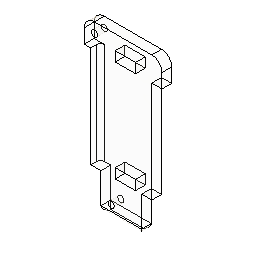
HolderThrower v5 (Autodesk Fusion 360 design; units mm, degrees)
Autodesk Fusion 360 part; units mm, degrees
sketch "Sketch1" plane through (0, 0, 0) normal (0, 1, 0) x (1, 0, 0)
  circle A0 centre (0, 0) radius 14 construction
  circle A1 centre (0, 0) radius 48 construction
  circle A2 centre (0, 0) radius 58 construction
  circle A3 centre (0, 0) radius 68 construction
  line L0 (0, 0) -> (0, 52) construction
  line L1 (-9.7468, 47) -> (-49.1426, 47) construction
  line L2 (-35.0918, 32.75) -> (-59.5939, 32.75) construction
  line L3 (-39.023, 27.95) -> (-61.9903, 27.95) construction
  line L4 (-42.7385, -21.85) -> (-64.3939, -21.85) construction
  circle A4 centre (-50.3158, -28.85) radius 1.5
  circle A5 centre (-42.1187, 39.875) radius 1.5
  line L5 (-55.3158, -21.85) -> (-55.3158, -28.85)
  line L6 (-50.3158, -33.85) -> (-22.1187, -33.85)
  line L7 (-22.1187, -21.85) -> (-22.1187, 27.95)
  line L8 (-27.1187, 44.875) -> (-47.1187, 44.875)
  line L9 (-52.1187, -21.85) -> (-55.3158, -21.85)
  line L10 (-30.1187, 27.95) -> (-40.1187, 27.95)
  arc A6 (-50.3158, -33.85) -> (-55.3158, -28.85) centre (-50.3158, -28.85) ccw construction
  arc A7 (-55.3158, -28.85) -> (-50.3158, -33.85) centre (-50.3158, -28.85) ccw
  line L11 (-55.3158, -33.85) -> (-50.3158, -33.85) construction
  line L12 (-55.3158, -28.85) -> (-55.3158, -33.85) construction
  line L13 (-22.1187, -21.85) -> (-17.1187, -21.85)
  line L14 (-17.1187, -21.85) -> (-17.1187, -28.85)
  line L15 (-22.1187, -33.85) -> (-17.1187, -33.85) construction
  line L16 (-17.1187, -28.85) -> (-17.1187, -33.85) construction
  arc A8 (-17.1187, -28.85) -> (-22.1187, -33.85) centre (-22.1187, -28.85) ccw construction
  arc A9 (-22.1187, -33.85) -> (-17.1187, -28.85) centre (-22.1187, -28.85) ccw
  line L17 (-65.8278, -17.05) -> (-44.8698, -17.05) construction
  line L18 (-40.1187, -21.85) -> (-30.1187, -21.85)
  line L19 (-30.1187, -21.85) -> (-30.1187, -26.65)
  line L20 (-30.1187, -26.65) -> (-40.1187, -26.65)
  line L21 (-40.1187, -26.65) -> (-40.1187, -21.85)
  line L22 (-40.1187, 27.95) -> (-40.1187, 23.15)
  line L23 (-40.1187, 23.15) -> (-30.1187, 23.15)
  line L24 (-30.1187, 23.15) -> (-30.1187, 27.95)
  line L25 (-30.1187, -21.85) -> (-22.1187, -21.85) construction
  line L26 (-52.1187, 27.95) -> (-47.1187, 27.95)
  line L27 (-47.1187, 27.95) -> (-47.1187, 44.875)
  line L28 (-22.1187, 27.95) -> (-27.1187, 27.95)
  line L29 (-27.1187, 27.95) -> (-27.1187, 44.875)
  line L30 (-27.1187, 27.95) -> (-30.1187, 27.95) construction
  line L31 (-52.1187, 27.95) -> (-52.1187, -21.85)
  point P0 (0, 14)
  point P1 (-42.1187, 39.875)
  point P2 (-50.3158, -28.85)
  dimension "d1" = 28
  dimension "d2" = 96
  dimension "d3" = 116
  dimension "d4" = 136
  dimension "d5" = 38
  dimension "d6" = 5
  dimension "d7" = 19.25
  dimension "d8" = 4.8
  dimension "d11" = 7
  dimension "d12" = 7.125
  dimension "d13" = 3
  dimension "d14" = 3
  dimension "d15" = 10
  dimension "d24" = 5
  dimension "d27" = 5
  dimension "d28" = 10
  dimension "d29" = 4.8
  dimension "d30" = 45
  dimension "d31" = 10
  dimension "d32" = 4.8
  dimension "d34" = 8
  dimension "d35" = 4.8
  dimension "d36" = 10
  dimension "d37" = 8
  dimension "d38" = 5
  dimension "d39" = 5
  dimension "d40" = 5
  dimension "d43" = 12
  constraint coincident A0.centre A1.centre
  constraint concentric A0 A1
  constraint concentric A1 A2
  constraint concentric A0 A3
  constraint vertical L0
  constraint coincident L0 P0
  constraint coincident A0 P0
  constraint coincident A1 L1.start
  constraint coincident A3 L1.end
  constraint horizontal L1
  constraint coincident A1 L2.start
  constraint coincident A3 L2.end
  constraint parallel L1 L2
  constraint coincident A1 L3.start
  constraint coincident A3 L3.end
  constraint parallel L2 L3
  constraint coincident A1 L4.start
  constraint coincident A3 L4.end
  constraint coincident A2 P1
  constraint coincident A2 P2
  constraint coincident P2 A4.centre
  constraint coincident P1 A5.centre
  constraint coincident L4 L5.start
  constraint perpendicular L4 L5
  constraint perpendicular L5 L6
  constraint perpendicular L6 L7
  constraint perpendicular L7 L8
  constraint coincident L4 L9.start
  constraint concentric A4 A6
  constraint tangent L5 A6
  constraint tangent L6 A6
  constraint horizontal L10
  constraint concentric A6 A7
  constraint perpendicular L5 L11
  constraint perpendicular L4 L12
  constraint perpendicular L7 L13
  constraint perpendicular L13 L14
  constraint tangent L6 A8
  constraint tangent L14 A8
  constraint perpendicular L5 L15
  constraint perpendicular L13 L16
  constraint concentric A8 A9
  constraint coincident A3 L17.start
  constraint coincident A1 L17.end
  constraint horizontal L18
  constraint vertical L19
  constraint horizontal L20
  constraint vertical L21
  constraint coincident L4 L18.start
  constraint perpendicular L10 L22
  constraint perpendicular L22 L23
  constraint perpendicular L10 L24
  constraint perpendicular L7 L25
  constraint collinear L3 L10
  constraint coincident L3 L26.start
  constraint perpendicular L8 L27
  constraint perpendicular L7 L28
  constraint perpendicular L8 L29
  constraint perpendicular L24 L30
  constraint perpendicular L26 L31
  constraint parallel L27 L31
  measures "d1" diameter of A0
  measures "d2" diameter of A1
  measures "d3" diameter of A2
  measures "d4" diameter of A3
  measures "d5" distance of L0.end P0
  measures "d6" distance of L0.end L1
  measures "d7" distance of L0.end L2
  measures "d8" distance of L2 L3
  measures "d11" distance of L4 P2
  measures "d12" distance of L2 P1
  measures "d13" diameter of A4
  measures "d14" diameter of A5
  measures "d15" diameter of A6
  measures "d24" distance of P1 L8
  measures "d27" distance of L7.start L13.end
  measures "d28" diameter of A8
  measures "d29" distance of L4 L17
  measures "d30" distance of L3 L17
  measures "d31" distance of L18.start L18.end
  measures "d32" distance of L18.start L20.end
  measures "d34" distance of L7 L19
  measures "d35" distance of L10.end L22.end
  measures "d36" distance of L22.end L23.end
  measures "d37" distance of L7 L24
  measures "d38" distance of L26.start L26.end
  measures "d39" distance of L7.end L28.end
  measures "d40" distance of P1 L27
  measures "d43" distance of L22 L31
extrude "Extrude1" add sketch "Sketch1" along normal blind 4.8
fillet "Fillet1" radius 2 4 edges at (-37.1187, 0, -44.875) (-47.1187, 2.4, -44.875) (-37.1187, 4.8, -44.875) (-27.1187, 2.4, -44.875)
fillet "Fillet2" radius 2 1 edges at (-52.1187, 4.8, -3.05)
